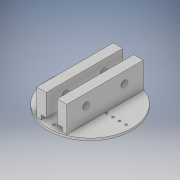
# Autodesk Inventor part: horn_fin_normal
Saved by Autodesk Inventor 2019 (Build 230136000, 136)
## iProperties
Created: 2020-07-18
Part Number: horn_fin_normal
Material: Generic
Document SubType Name: Modeling
Designer: Agus Prayudi
Density: 1 g/cm^3
Appearance: Default
Author: Agus Prayudi
Autodesk Inventor part; units mm, degrees
ref_plane "XZ Plane" through (0, 0, 0) normal (0, 1, 0) x (-1, 0, 0)
sketch "Sketch1" plane through (0, 0, 0) normal (0, 1, 0) x (-1, 0, 0)
  circle A0 centre (0, 27.06) radius 0.5
  circle A1 centre (0, 24.06) radius 0.5
  circle A2 centre (0, 16.53) radius 4.375
  circle A3 centre (0, 3) radius 0.5
  circle A4 centre (0, 6) radius 0.5
  circle A5 centre (0, 9) radius 0.5
  circle A6 centre (0, 0) radius 0.5
  circle A7 centre (0, 30.06) radius 0.5
  circle A8 centre (0, 33.06) radius 0.5
  circle A9 centre (0, 16.53) radius 19.18
  constraints: 10 centre point, 1 coincident
extrude "Extrusion1" add sketch "Sketch1" along normal blind 1
sketch "Sketch5" plane through (0, 1, 16.53) normal (0, 1, 0) x (1, 0, 0)
  line L0 (4.875, 0) -> (4.875, -17.5)
  line L1 (4.875, -17.5) -> (6.875, -17.5)
  line L2 (6.875, -17.5) -> (6.875, 0)
  line L3 (4.875, 0) -> (4.875, 17.5)
  line L4 (4.875, 17.5) -> (6.875, 17.5)
  line L5 (6.875, 17.5) -> (6.875, 0)
  point P0 (0, 16.53)
  constraints: 12 end point, 2 perpendicular
extrude "Extrusion4" add sketch "Sketch5" along normal blind 12
sketch "Sketch6" plane through (4.875, 1, -0.97) normal (-1, 0, 0) x (0, 0, 1)
  line L0 (36.68, 0) -> (-1.68, 0) projected
  line L1 (35, 2) -> (17.5, 2)
  line L2 (17.5, 2) -> (0, 2)
  line L3 (0, 12) -> (35, 12)
  line L4 (35, 2) -> (35, 12)
  line L5 (0, 2) -> (0, 12)
  circle A0 centre (8.75, 7) radius 1.5
  circle A1 centre (26.25, 7) radius 1.5
  point P0 (0.97, -1)
  dimension "d18" = 3
  constraints: 10 end point, 2 centre point, 1 horizontal, 1 perpendicular, 1 point on line
  measures "d18" diameter of A0
extrude "Extrusion5" cut sketch "Sketch6" against normal blind 12 contours A0 | A1
extrude "Extrusion6" add sketch "Sketch6" along normal blind 2.375
ref_plane "Work Plane1" through (0, 0, 0) normal (1, 0, 0) x (0, 1, 0)
mirror "Mirror1" about plane through (0, 0, 0) normal (1, 0, 0) of "Extrusion6", "Extrusion4", "Extrusion5"
ref_plane "Work Plane2" through (0, 1, 16.53) normal (0, 1, 0) x (1, 0, 0)
sketch "Sketch7" plane through (0, 1, 16.53) normal (0, 1, 0) x (1, 0, 0)
  circle A0 centre (0, 0) radius 4.375 projected
  circle A1 centre (0, 16.53) radius 0.5 projected
  circle A2 centre (0, 13.53) radius 0.5 projected
  circle A3 centre (0, 10.53) radius 0.5 projected
  circle A4 centre (0, 7.53) radius 0.5 projected
  circle A5 centre (0, -10.53) radius 0.5 projected
  circle A6 centre (0, -16.53) radius 0.5 projected
  circle A7 centre (0, -13.53) radius 0.5 projected
  circle A8 centre (0, -7.53) radius 0.5 projected
  circle A9 centre (0, 0) radius 19.18 projected
  circle A10 centre (0, 0) radius 4.375 projected
  circle A11 centre (7.53, 0) radius 0.5
  circle A12 centre (10.53, 0) radius 0.5
  circle A13 centre (13.53, 0) radius 0.5
  circle A14 centre (16.53, 0) radius 0.5
  circle A15 centre (0, -13.53) radius 0.5
  circle A16 centre (-7.53, 0) radius 0.5
  circle A17 centre (-10.53, 0) radius 0.5
  circle A18 centre (-13.53, 0) radius 0.5
  circle A19 centre (-16.53, 0) radius 0.5
  constraints: 9 centre point
extrude "Extrusion7" cut sketch "Sketch7" along normal mid plane 10 contours A11 | A12 | A13 | A14 | A16 | A17 | A18 | A19
body "Solid1"
